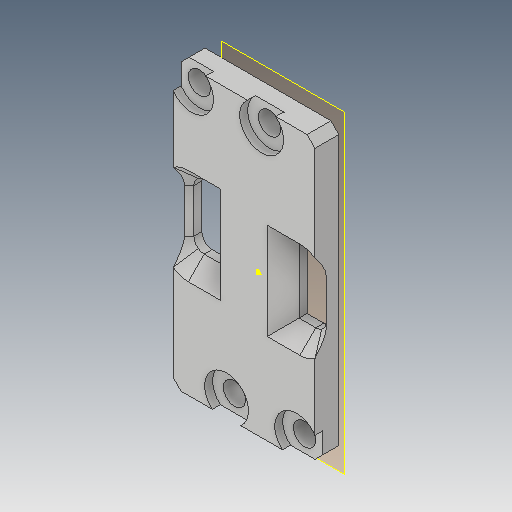
# Autodesk Inventor part: 02_Camera_Module_Lid_v0
Saved by Autodesk Inventor 2019 (Build 230136000, 136)
## iProperties
Created: 2021-09-09
Part Number: 02_Camera_Module_Lid_v0
Material: Generisch
Document SubType Name: Modeling
Designer: Muriel
Density: 1 g/cm^3
Appearance: Vorgabe
Author: Muriel
Autodesk Inventor part; units mm, degrees
note: some values were not read from the file. Chosen so that the rebuilt part matches the saved one: sketch regions of "Extrusion1".
ref_plane "YZ Plane" through (0, 0, 0) normal (1, 0, 0) x (0, 1, 0)
ref_plane "XZ Plane" through (0, 0, 0) normal (0, 1, 0) x (-1, 0, 0)
ref_plane "XY Plane" through (0, 0, 0) normal (0, 0, 1) x (1, 0, 0)
ref_plane "Arbeitsebene1" through (0, 0, 0) normal (0, 0, 1) x (1, 0, 0)
sketch "Skizze1" plane through (0, 0, 0) normal (0, 0, 1) x (1, 0, 0)
  line L0 (6, 17.9) -> (7, 16.9) projected
  line L1 (3.1, 17.9) -> (6, 17.9) projected
  line L2 (3.1, 14) -> (3.1, 17.9) projected
  line L3 (3.5, 14) -> (3.1, 14) projected
  line L4 (3.5, 10) -> (3.5, 14) projected
  line L5 (6.4, 10) -> (3.5, 10) projected
  line L6 (6.4, -11.4) -> (6.4, 10) projected
  line L7 (3.8, -11.4) -> (6.4, -11.4) projected
  line L8 (3.8, -14.4) -> (3.8, -11.4) projected
  line L9 (1.3, -14.4) -> (3.8, -14.4) projected
  line L10 (1.3, -13.4) -> (1.3, -14.4) projected
  line L11 (-0.7, -13.4) -> (1.3, -13.4) projected
  line L12 (-0.7, -14.4) -> (-0.7, -13.4) projected
  line L13 (-6.9, -14.4) -> (-5.1, -14.4) projected
  line L14 (-4.1, -13.4) -> (-4.1, -14.4) projected
  line L15 (-5.1, -13.4) -> (-4.1, -13.4) projected
  line L16 (-5.1, -14.4) -> (-5.1, -13.4) projected
  line L17 (-6.9, -17.9) -> (-6.9, -14.4) projected
  line L18 (6, -17.9) -> (-6.9, -17.9) projected
  line L19 (7, -16.9) -> (6, -17.9) projected
  line L20 (7, 16.9) -> (7, -16.9) projected
  line L21 (6, 17.9) -> (7, 16.9) projected
  line L22 (3.1, 17.9) -> (6, 17.9) projected
  line L23 (3.1, 14) -> (3.1, 17.9) projected
  line L24 (3.5, 14) -> (3.1, 14) projected
  line L25 (3.5, 10) -> (3.5, 14) projected
  line L26 (6.4, 10) -> (3.5, 10) projected
  line L27 (6.4, -11.4) -> (6.4, 10) projected
  line L28 (3.8, -11.4) -> (6.4, -11.4) projected
  line L29 (3.8, -14.4) -> (3.8, -11.4) projected
  line L30 (1.3, -14.4) -> (3.8, -14.4) projected
  line L31 (1.3, -13.4) -> (1.3, -14.4) projected
  line L32 (-0.7, -13.4) -> (1.3, -13.4) projected
  line L33 (-0.7, -14.4) -> (-0.7, -13.4) projected
  line L34 (-6.9, -14.4) -> (-5.1, -14.4) projected
  line L35 (-4.1, -13.4) -> (-4.1, -14.4) projected
  line L36 (-5.1, -13.4) -> (-4.1, -13.4) projected
  line L37 (-5.1, -14.4) -> (-5.1, -13.4) projected
  line L38 (-6.9, -17.9) -> (-6.9, -14.4) projected
  line L39 (6, -17.9) -> (-6.9, -17.9) projected
  line L40 (7, -16.9) -> (6, -17.9) projected
  line L41 (7, 16.9) -> (7, -16.9) projected
  line L42 (-9.8, -17.9) -> (-10.8, -16.9) projected
  line L43 (-6.9, -17.9) -> (-9.8, -17.9) projected
  line L44 (-6.9, -14) -> (-6.9, -17.9) projected
  line L45 (-7.3, -14) -> (-6.9, -14) projected
  line L46 (-7.3, -10) -> (-7.3, -14) projected
  line L47 (-10.2, -10) -> (-7.3, -10) projected
  line L48 (-10.2, 11.4) -> (-10.2, -10) projected
  line L49 (-7.6, 11.4) -> (-10.2, 11.4) projected
  line L50 (-7.6, 14.4) -> (-7.6, 11.4) projected
  line L51 (-5.1, 14.4) -> (-7.6, 14.4) projected
  line L52 (-5.1, 13.4) -> (-5.1, 14.4) projected
  line L53 (-3.1, 13.4) -> (-5.1, 13.4) projected
  line L54 (-3.1, 14.4) -> (-3.1, 13.4) projected
  line L55 (3.1, 14.4) -> (1.3, 14.4) projected
  line L56 (0.3, 13.4) -> (0.3, 14.4) projected
  line L57 (1.3, 13.4) -> (0.3, 13.4) projected
  line L58 (1.3, 14.4) -> (1.3, 13.4) projected
  line L59 (3.1, 17.9) -> (3.1, 14.4) projected
  line L60 (-9.8, 17.9) -> (3.1, 17.9) projected
  line L61 (-10.8, 16.9) -> (-9.8, 17.9) projected
  line L62 (-10.8, -16.9) -> (-10.8, 16.9) projected
  arc A0 (5.1, -4.25) -> (6.1, -3.25) centre (5.1, -3.25) ccw construction
  line L63 (6.1, 2.25) -> (6.1, -3.25) construction
  arc A1 (6.1, 2.25) -> (5.1, 3.25) centre (5.1, 2.25) ccw construction
  line L64 (3.3, 3.25) -> (5.1, 3.25) construction
  line L65 (3.3, 3.25) -> (3.3, -4.25) construction
  line L66 (3.3, -4.25) -> (5.1, -4.25) construction
  arc A2 (-8.9, 4.25) -> (-9.9, 3.25) centre (-8.9, 3.25) ccw construction
  line L67 (-9.9, -2.25) -> (-9.9, 3.25) construction
  arc A3 (-9.9, -2.25) -> (-8.9, -3.25) centre (-8.9, -2.25) ccw construction
  line L68 (-7.1, -3.25) -> (-8.9, -3.25) construction
  line L69 (-7.1, -3.25) -> (-7.1, 4.25) construction
  line L70 (-7.1, 4.25) -> (-8.9, 4.25) construction
  line L71 (3, -4.55) -> (3, 3.55)
  line L72 (3, 3.55) -> (5.1, 3.55)
  arc A4 (6.4, 2.25) -> (5.1, 3.55) centre (5.1, 2.25) ccw
  line L73 (6.4, 2.25) -> (6.4, -3.25)
  arc A5 (5.1, -4.55) -> (6.4, -3.25) centre (5.1, -3.25) ccw
  line L74 (5.1, -4.55) -> (3, -4.55)
  arc A6 (-10.2, -2.25) -> (-8.9, -3.55) centre (-8.9, -2.25) ccw
  line L75 (-10.2, -2.25) -> (-10.2, 3.25)
  arc A7 (-8.9, 4.55) -> (-10.2, 3.25) centre (-8.9, 3.25) ccw
  line L76 (-8.9, 4.55) -> (-6.8, 4.55)
  line L77 (-6.8, 4.55) -> (-6.8, -3.55)
  line L78 (-6.8, -3.55) -> (-8.9, -3.55)
  circle A8 centre (4.7, -15.8) radius 1.4 projected
  circle A9 centre (4.7, -15.8) radius 1.4 projected
  circle A10 centre (-8.5, 15.8) radius 1.4 projected
  circle A11 centre (-4.1, -15.8) radius 1.4 projected
  circle A12 centre (-4.1, -15.8) radius 1.4 projected
  line L79 (-4.1, -14.4) -> (-0.7, -14.4) projected
  circle A13 centre (-4.1, -15.8) radius 1.4 projected
  circle A14 centre (-4.1, -15.8) radius 1.4 projected
  line L80 (-4.1, -14.4) -> (-0.7, -14.4) projected
  circle A15 centre (0.3, 15.8) radius 1.4 projected
  circle A16 centre (0.3, 15.8) radius 1.4 projected
  line L81 (0.3, 14.4) -> (-3.1, 14.4) projected
  point P0 (0, 0)
  point P1 (-2.4, -14.4)
  point P2 (-2.5, -14.4)
  point P3 (-1.4, 14.4)
  point P4 (-1.3, 14.4)
  dimension "d0" = 0.3
  dimension "d1" = 0.3
  constraints: 16 end point, 8 point on circle, 6 vertical alignment, 4 centre point, 10 other
  measures "d0" distance between parallel lines of L65 L71
  measures "d1" radial gap between concentric circles of A3 A6
extrude "Extrusion1" add sketch "Skizze1" along normal blind 3 contours A11 | L0 L20 L19 L18 L17 L13 L16 L15 L14 L79 L12 L11 L10 L9 L8 L7 L6 L5 L4 L3 L2 L1 | A15 | L2 L55 L58 L57 L56 L81 L54 L53 L52 L51 L50 L49 L48 L47 L46 L45 L44 L17 L43 L42 L62 L61 L60 | L2 L3 L4 L5 L6 A4 L72 L71 L74 A5 L7 L8 L9 L10 L11 L12 L79 L14 L15 L16 L13 L44 L45 L46 L47 L48 A6 L78 L77 L76 A7 L49 L50 L51 L52 L53 L54 L81 L56 L57 L58 L55 | A8 | A10
sketch "Skizze2" plane through (0, 0, 3) normal (0, 0, 1) x (1, 0, 0)
  point P0 (0, 0)
sketch "Skizze3" plane through (0, 0, 3) normal (0, 0, 1) x (1, 0, 0)
  circle A0 centre (-8.5, 15.8) radius 1.4 projected
  circle A1 centre (0.3, 15.8) radius 1.4 projected
  circle A2 centre (4.7, -15.8) radius 1.4 projected
  circle A3 centre (-4.1, -15.8) radius 1.4 projected
  point P0 (0, 0)
  constraints: 1 coincident
hole "Bohrung1" at (0.3, 15.8, 3) at (4.7, -15.8, 3) at (-4.1, -15.8, 3) at (-8.5, 15.8, 3) direction (0, 0, -1) diameter 2.8 depth 12 tip angle 118 counterbore diameter 5.5 counterbore depth 1
chamfer "Fase1" distance 2 angle 45 12 edges at (6.0192, 3.1692, 3) (6.4, -0.5, 3) (6.0192, -4.1692, 3) (4.05, -4.55, 3) (4.05, 3.55, 3) (3, -0.5, 3) (-6.8, 0.5, 3) (-9.8192, 4.1692, 3) (-7.85, 4.55, 3) (-10.2, 0.5, 3) (-9.8192, -3.1692, 3) (-7.85, -3.55, 3)
